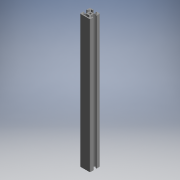
# Autodesk Inventor part: NFSF5-2020-263.5
Saved by Autodesk Inventor 2017.3 (Build 213256000, 256)
## iProperties
Part Number: NFSF5-2020-263.5
Material: Generic
Catalog Web Link: www.cadenas.de
Description: NFS5-2020, NFSB5-2020, HFS5-2020, HFSB5-2020, CAF5-2020, HFSY5-2020, NFSF5-2020, HFSF5-2020, HFSFB5-2020, NFST5-2020, HFST5-2020, HFSTB5-2020, HFSH5-2020, HFSC5-2020-HFS5 Series Aluminum Extrusions 20 Square -1 Slot-
Vendor: MISUMI
Document SubType Name: Modeling
Designer: partserver
Manufacturer: MISUMI
Mass: 51.0572 g
Surface Area: 481.65 cm^2
Volume: 51.0572 cm^3
Density: 1 g/cm^3
Appearance: PSOLRGB-175-175-175
Category: PARTsolutions
Company: MISUMI
Title: NFSF5-2020-263.5
Author: Cadenas PARTsolutions
Comments: HFS5 Series Aluminum Extrusions 20 Square -1 Slot-
PSOL_IDENT_0: {$CADENAS_DATA\23d-libs\misumi\metric\38_al_extrusions_blackets\5\hfs5_2020.prj},682 {VTYP=3D},{NB=N
PSOL_IDENT_1: FSF5-2020-263.5},{LINA=NFSF5-2020-263.5},{NN=NFS5-2020, NFSB5-2020, HFS5-2020, HFSB5-2020, CAF5-2020
PSOL_IDENT_2: , HFSY5-2020, NFSF5-2020, HFSF5-2020, HFSFB5-2020, NFST5-2020, HFST5-2020, HFSTB5-2020, HFSH5-2020,
PSOL_IDENT_3: HFSC5-2020},{DATE=09.09.2019 15:28:27},{GEOMDATE=18.06.2019 07:59:14},{VERSION=},{LINEID=40},{WBVAR=
PSOL_IDENT_4: L,ALT1,ALT2,ALT4,ALT5,CP5,DL5,DR5,ALT6,ALT9,ALT10,ALT11,HP6,NHL6,DL6,NHR6,DR6,ALT7,ALT8,NH9,AH,BH,CH
PSOL_IDENT_5: ,DH,EH,NH10,AV,BV,CV,DV,EV,NH11,AP,BP,CP,DP,EP,ALT12,ALT13,Z,NH12,XA,XB,XC,XD,XE,NH13,YA,YB,YC,YD,YE
PSOL_IDENT_6: ,ALT16,HP16,DL16,DR16,ALT17,HQ17,JLP,ALT20},{WBNUMERIC=L,NH9,AH,BH,CH,DH,EH,NH10,AV,BV,CV,DV,EV,NH11
PSOL_IDENT_7: ,AP,BP,CP,DP,EP,NH12,XA,XB,XC,XD,XE,NH13,YA,YB,YC,YD,YE,HQ17,JLP}  {NB=NFSF5-2020-263.5},{LINA=NFSF5
PSOL_IDENT_8: -2020-263.5},{KT=DUMMY},{PN=NFSF5-2020-263.5},{TPS=NFSF5-2020},{MAT=6063-T5 Aluminum Alloy},{ST=Clea
PSOL_IDENT_9: r Anodize},{FRMW=20},{FRMH=20},{FRD=4.2},{L=263.5},{MASS=0.53},{SA=195},{LX=0.834x10^4},{LY=0.746x10
PSOL_IDENT_10: ^4},{ALT1=},{M1=0},{DPL1=0},{DPR1=0},{ALT1PN=},{ALT2=},{ALT2ALG= '','w/o End Tapping (Heli-Coil Inse
PSOL_IDENT_11: rt)','LHP','with LHP (Tapping on the Left (Heli-Coil Insert))','RHP','with RHP (Tapping on the Right
PSOL_IDENT_12: (Heli-Coil Insert))','HPW','with HPW (Tapping on Both Ends (Heli-Coil Insert))' },{M2=0},{DP2=0},{A
PSOL_IDENT_13: LT2PN=},{ALT4=},{ALT4ALG= '', 'w/o SC (High Precision Cut)', 'SC', 'with SC (High Precision Cut)' },
PSOL_IDENT_14: {ALT4PN=},{ALT5=},{ALT5ALG= '','w/o 45 Degree Cut','1','with 45 Degree Cut' },{CP5=},{CP5ALG= '','N/
PSOL_IDENT_15: A' },{DL5=},{DL5ALG= '','N/A' },{DR5=},{DR5ALG= '','N/A' },{FRMLALT5=0},{FRMRALT5=0},{ALT5PN=},{ALT6=
PSOL_IDENT_16: },{ALT6ALG= '','w/o Fastening Location Wrench Access Hole Alterations','1','with Fastening Location
PSOL_IDENT_17: Wrench Access Hole Alterations' },{ALT9=},{ALT9ALG= '','w/o Location Specified Wrench Access Hole Al
PSOL_IDENT_18: teratons (Horizontal)','1','with Location Specified Wrench Access Hole Alteratons (Horizontal)' },{A
PSOL_IDENT_19: LT10=},{ALT10ALG= '','w/o Location Specified Wrench Access Hole Alteratons (Vertical)','1','with Loc
PSOL_IDENT_20: ation Specified Wrench Access Hole Alteratons (Vertical)' },{ALT11=},{ALT11ALG= '','w/o Location Spe
PSOL_IDENT_21: cified Wrench Access Hole Alteratons (Crisscross)','1','with Location Specified Wrench Access Hole A
PSOL_IDENT_22: lteratons (Crisscross)' },{HP6=},{HP6ALG= '','N/A' },{NHL6=},{NHL6ALG= '','N/A' },{DL6=},{DL6ALG= ''
PSOL_IDENT_23: ,'N/A' },{NHR6=},{NHR6ALG= '','N/A' },{DR6=},{DR6ALG= '','N/A' },{HL6=0.000},{HL6D=0},{HR6=0.000},{H
PSOL_IDENT_24: R6D=0},{J6=0},{J6D=0},{K6=0},{K6D=0},{DD6=0.00},{DD6ALG=0},{ALT7=},{ALT7ALG= '','N/A' },{ALT8=},{ALT
PSOL_IDENT_25: 8ALG= '','N/A' },{ALT678PN=},{NH9=0},{NH9MAX=5},{NH9ALG=[0]},{AH=0.0},{AHMIN=7},{AHMAX=258.5},{AHALG=
PSOL_IDENT_26: [0]},{BH=0.0},{BHMIN=2},{BHMAX=260.5},{BHALG=[0]},{CH=0.0},{CHMIN=2},{CHMAX=262.5},{CHALG=[0]},{DH=0
PSOL_IDENT_27: .0},{DHMIN=2},{DHMAX=264.5},{DHALG=[0]},{EH=0.0},{EHMIN=2},{EHMAX=256.5},{EHALG=[0]},{NH10=0},{NH10M
PSOL_IDENT_28: AX=5},{NH10ALG=[0]},{AV=0.0},{AVMIN=7},{AVMAX=258.5},{AVALG=[0]},{BV=0.0},{BVMIN=2},{BVMAX=260.5},{B
PSOL_IDENT_29: VALG=[0]},{CV=0.0},{CVMIN=2},{CVMAX=262.5},{CVALG=[0]},{DV=0.0},{DVMIN=2},{DVMAX=264.5},{DVALG=[0]},
PSOL_IDENT_30: {EV=0.0},{EVMIN=2},{EVMAX=256.5},{EVALG=[0]},{NH11=0},{NH11MAX=5},{NH11ALG=[0]},{AP=0.0},{APMIN=7},{
PSOL_IDENT_31: APMAX=258.5},{APALG=[0]},{BP=0.0},{BPMIN=2},{BPMAX=260.5},{BPALG=[0]},{CP=0.0},{CPMIN=2},{CPMAX=262.
PSOL_IDENT_32: 5},{CPALG=[0]},{DP=0.0},{DPMIN=2},{DPMAX=264.5},{DPALG=[0]},{EP=0.0},{EPMIN=2},{EPMAX=256.5},{EPALG=
PSOL_IDENT_33: [0]},{ALT9PN=},{ALT10PN=},{ALT11PN=},{ALT91011PN=},{ALT12=},{ALT12ALG= '','w/o Counterbore Hole in S
PSOL_IDENT_34: pecified Position (Vertical)','1','with Counterbore Hole in Specified Position (Vertical)' },{ALT13=
PSOL_IDENT_35: },{ALT13ALG= '','w/o Counterbore Hole in Specified Position (Horizontal)','1','with Counterbore Hole
PSOL_IDENT_36: in Specified Position (Horizontal)' },{Z=},{ZALG= '','N/A' },{DD12=0.0},{DD112=0.0},{NH12=0},{NH12M
PSOL_IDENT_37: AX=5},{NH12ALG=[0]},{XA=0.0},{XAMIN=7},{XAMAX=258.5},{XAALG=[0]},{XB=0.0},{XBMIN=2},{XBMAX=260.5},{X
PSOL_IDENT_38: BALG=[0]},{XC=0.0},{XCMIN=2},{XCMAX=262.5},{XCALG=[0]},{XD=0.0},{XDMIN=2},{XDMAX=264.5},{XDALG=[0]},
PSOL_IDENT_39: {XE=0.0},{XEMIN=2},{XEMAX=256.5},{XEALG=[0]},{NH13=0},{NH13MAX=5},{NH13ALG=[0]},{YA=0.0},{YAMIN=7},{
PSOL_IDENT_40: YAMAX=258.5},{YAALG=[0]},{YB=0.0},{YBMIN=2},{YBMAX=260.5},{YBALG=[0]},{YC=0.0},{YCMIN=2},{YCMAX=262.
PSOL_IDENT_41: 5},{YCALG=[0]},{YD=0.0},{YDMIN=2},{YDMAX=264.5},{YDALG=[0]},{YE=0.0},{YEMIN=2},{YEMAX=256.5},{YEALG=
PSOL_IDENT_42: [0]},{ALT12PN=},{ALT13PN=},{ALT1213PN=},{ALT16=},{ALT16ALG= '','w/o M Type Hole Alteration','1','wit
PSOL_IDENT_43: h M Type Hole Alteration' },{HP16=},{HP16ALG= '','N/A' },{DL16=},{DL16ALG= '','N/A' },{DR16=},{DR16A
PSOL_IDENT_44: LG= '','N/A' },{H116=0},{D16=0.0},{ALT16PN=},{ALT17=},{ALT17ALG= '','w/o L Type Hole Alteration (Top
PSOL_IDENT_45: )','1','with L Type Hole Alteration (Top)' },{HQ17=0},{HQ17ALG=0},{JLP=0},{JLPMIN=4.9},{JLPMAX=0},{J
PSOL_IDENT_46: LPALG=[0]},{L17=0},{D17=0.0},{ALT17PN=},{ALT20=},{ALT20PN=},{ERRORALT01=OK},{ERRORALT02=OK},{ERRORAL
PSOL_IDENT_47: T05=OK},{ERRORALT06091=OK},{ERRORALT06092=OK},{ERRORALT06093=OK},{ERRORALT06094=OK},{ERRORALT06101=O
PSOL_IDENT_48: K},{ERRORALT06102=OK},{ERRORALT06103=OK},{ERRORALT06104=OK},{ERRORALT06111=OK},{ERRORALT06112=OK},{E
PSOL_IDENT_49: RRORALT06113=OK},{ERRORALT06114=OK},{ERRORALT06121=OK},{ERRORALT06122=OK},{ERRORALT06123=OK},{ERRORA
PSOL_IDENT_50: LT06124=OK},{ERRORALT06131=OK},{ERRORALT06132=OK},{ERRORALT06133=OK},{ERRORALT06134=OK},{ERRORALT061
PSOL_IDENT_51: 6=OK},{ERRORALT06171=OK},{ERRORALT06172=OK},{ERRORALT06173=OK},{ERRORALT0911=OK},{ERRORALT0913=OK},{
PSOL_IDENT_52: ERRORALT0916=OK},{ERRORALT0917=OK},{ERRORALT1011=OK},{ERRORALT1012=OK},{ERRORALT1016=OK},{ERRORALT10
PSOL_IDENT_53: 17=OK},{ERRORALT1112=OK},{ERRORALT1113=OK},{ERRORALT1116=OK},{ERRORALT1117=OK},{ERRORALT1216=OK},{ER
PSOL_IDENT_54: RORALT1217=OK},{ERRORALT1316=OK},{ERRORALT1317=OK},{ERRORALT1617=OK},{ERRORPN=},{TFW=0}
NB: NFSF5-2020-263.5
NN: NFS5-2020, NFSB5-2020, HFS5-2020, HFSB5-2020, CAF5-2020, HFSY5-2020, NFSF5-2020, HFSF5-2020, HFSFB5-2020, NFST5-2020, HFST5-2020, HFSTB5-2020, HFSH5-2020, HFSC5-2020
NT: HFS5 Series Aluminum Extrusions 20 Square -1 Slot-
NBSYN: $PN.
LINA: NFSF5-2020-263.5
CATALOG: Misumi
PN: NFSF5-2020-263.5
TPS: NFSF5-2020
MAT: 6063-T5 Aluminum Alloy
ST: Clear Anodize
L: 263.5
MASS: 0.53
SA: 195
LX: 0.834x10^4
LY: 0.746x10^4
ALT1: w/o End Tapping
M1: 0
DPL1: 0
DPR1: 0
ALT2: w/o End Tapping (Heli-Coil Insert)
M2: 0
DP2: 0
ALT4: w/o SC (High Precision Cut)
ALT5: w/o 45 Degree Cut
CP5: N/A
DL5: N/A
DR5: N/A
ALT6: w/o Fastening Location Wrench Access Hole Alterations
ALT9: w/o Location Specified Wrench Access Hole Alteratons (Horizontal)
ALT10: w/o Location Specified Wrench Access Hole Alteratons (Vertical)
ALT11: w/o Location Specified Wrench Access Hole Alteratons (Crisscross)
HP6: N/A
NHL6: N/A
DL6: N/A
NHR6: N/A
DR6: N/A
HL6D: 0
HR6D: 0
J6D: 0
K6D: 0
DD6: 0
ALT7: N/A
ALT8: N/A
NH9: 0
AH: 0
BH: 0
CH: 0
DH: 0
EH: 0
NH10: 0
AV: 0
BV: 0
CV: 0
DV: 0
EV: 0
NH11: 0
AP: 0
BP: 0
CP: 0
DP: 0
EP: 0
ALT12: w/o Counterbore Hole in Specified Position (Vertical)
ALT13: w/o Counterbore Hole in Specified Position (Horizontal)
Z: N/A
DD12: 0
DD112: 0
NH12: 0
XA: 0
XB: 0
XC: 0
XD: 0
XE: 0
NH13: 0
YA: 0
YB: 0
YC: 0
YD: 0
YE: 0
ALT16: w/o M Type Hole Alteration
HP16: N/A
DL16: N/A
DR16: N/A
H116: 0
D16: 0
ALT17: w/o L Type Hole Alteration (Top)
HQ17: 0
JLP: 0
D17: 0
ALT20: w/o CW (End Face C Chamfering)
SUPPLIER: MISUMI
ARTICLENO: NFSF5-2020-263.5
BOMINFO: NFSF5-2020-263.5
CREATOR: CADENAS GmbH
Autodesk Inventor part; units mm, degrees
ref_plane "YZ Plane" through (0, 0, 0) normal (1, 0, 0) x (0, 1, 0)
ref_plane "XZ Plane" through (0, 0, 0) normal (0, 1, 0) x (-1, 0, 0)
ref_plane "XY Plane" through (0, 0, 0) normal (0, 0, 1) x (1, 0, 0)
sketch "Sketch_76" plane through (0, 0, 0) normal (0, 0, 1) x (1, 0, 0)
  line L0 (-10, -3) -> (-10, -9)
  arc A0 (-10, -9) -> (-9, -10) centre (-9, -9) ccw
  line L1 (-9, -10) -> (9, -10)
  arc A1 (9, -10) -> (10, -9) centre (9, -9) ccw
  line L2 (10, -9) -> (10, -3)
  line L3 (10, -3) -> (8, -3)
  line L4 (8, -3) -> (8, -6)
  line L5 (8, -6) -> (7.0607, -6)
  line L6 (7.0607, -6) -> (4, -2.9393)
  line L7 (4, -2.9393) -> (4, -0.6536)
  arc A2 (4, -0.6536) -> (3.933, -0.4036) centre (3.5, -0.6536) ccw
  line L8 (3.933, -0.4036) -> (3.7, 0)
  line L9 (3.7, 0) -> (3.933, 0.4036)
  arc A3 (3.933, 0.4036) -> (3.933, 0.9036) centre (3.5, 0.6536) ccw
  line L10 (3.933, 0.9036) -> (3.751, 1.2189)
  line L11 (3.751, 1.2189) -> (4, 2.5)
  line L12 (4, 2.5) -> (4, 2.9393)
  line L13 (4, 2.9393) -> (7.0607, 6)
  line L14 (7.0607, 6) -> (8, 6)
  line L15 (8, 6) -> (8, 3)
  line L16 (8, 3) -> (10, 3)
  line L17 (10, 3) -> (10, 9)
  arc A4 (10, 9) -> (9, 10) centre (9, 9) ccw
  line L18 (9, 10) -> (3, 10)
  line L19 (3, 10) -> (3, 8)
  line L20 (3, 8) -> (6, 8)
  line L21 (6, 8) -> (6, 7.0607)
  line L22 (6, 7.0607) -> (2.9393, 4)
  line L23 (2.9393, 4) -> (0.6536, 4)
  arc A5 (0.6536, 4) -> (0.4036, 3.933) centre (0.6536, 3.5) ccw
  line L24 (0.4036, 3.933) -> (0, 3.7)
  line L25 (0, 3.7) -> (-0.4036, 3.933)
  arc A6 (-0.4036, 3.933) -> (-0.9036, 3.933) centre (-0.6536, 3.5) ccw
  line L26 (-0.9036, 3.933) -> (-1.2189, 3.751)
  line L27 (-1.2189, 3.751) -> (-2.5, 4)
  line L28 (-2.5, 4) -> (-2.9393, 4)
  line L29 (-2.9393, 4) -> (-6, 7.0607)
  line L30 (-6, 7.0607) -> (-6, 8)
  line L31 (-6, 8) -> (-3, 8)
  line L32 (-3, 8) -> (-3, 10)
  line L33 (-3, 10) -> (-9, 10)
  arc A7 (-9, 10) -> (-10, 9) centre (-9, 9) ccw
  line L34 (-10, 9) -> (-10, 3)
  line L35 (-10, 3) -> (-8, 3)
  line L36 (-8, 3) -> (-8, 6)
  line L37 (-8, 6) -> (-7.0607, 6)
  line L38 (-7.0607, 6) -> (-4, 2.9393)
  line L39 (-4, 2.9393) -> (-4, 0.6536)
  arc A8 (-4, 0.6536) -> (-3.933, 0.4036) centre (-3.5, 0.6536) ccw
  line L40 (-3.933, 0.4036) -> (-3.7, 0)
  line L41 (-3.7, 0) -> (-3.933, -0.4036)
  arc A9 (-3.933, -0.4036) -> (-3.933, -0.9036) centre (-3.5, -0.6536) ccw
  line L42 (-3.933, -0.9036) -> (-3.751, -1.2189)
  line L43 (-3.751, -1.2189) -> (-4, -2.5)
  line L44 (-4, -2.5) -> (-4, -2.9393)
  line L45 (-4, -2.9393) -> (-7.0607, -6)
  line L46 (-7.0607, -6) -> (-8, -6)
  line L47 (-8, -6) -> (-8, -3)
  line L48 (-8, -3) -> (-10, -3)
  line L49 (-6, -7.2678) -> (-6, -7.5)
  arc A10 (-6, -7.5) -> (-5.5, -8) centre (-5.5, -7.5) ccw
  line L50 (-5.5, -8) -> (5.5, -8)
  arc A11 (5.5, -8) -> (6, -7.5) centre (5.5, -7.5) ccw
  line L51 (6, -7.5) -> (6, -7.2678)
  arc A12 (6, -7.2678) -> (5.8536, -6.9142) centre (5.5, -7.2678) ccw
  line L52 (5.8536, -6.9142) -> (3.0858, -4.1464)
  arc A13 (3.0858, -4.1464) -> (2.7322, -4) centre (2.7322, -4.5) ccw
  line L53 (2.7322, -4) -> (-2.7322, -4)
  arc A14 (-2.7322, -4) -> (-3.0858, -4.1464) centre (-2.7322, -4.5) ccw
  line L54 (-3.0858, -4.1464) -> (-5.8536, -6.9142)
  arc A15 (-5.8536, -6.9142) -> (-6, -7.2678) centre (-5.5, -7.2678) ccw
  constraints: 110 end point, 32 point on circle, 16 centre point
extrude "Extrusion1" add sketch "Sketch_76" against normal blind 263.5
sketch "Sketch2" plane through (0, 0, -263.5) normal (0, 0, -1) x (-1, 0, 0)
  point P0 (0, 0)
hole "Hole1" at (0, 0, -263.5) direction (0, 0, 1) diameter 4.2 depth 263.5
ref_plane "C1_XY" through (0, 0, 0) normal (0, 0, 1) x (1, 0, 0)
ref_plane "C1_YZ" through (0, 0, 0) normal (1, 0, 0) x (0, 1, 0)
ref_plane "C1_ZX" through (0, 0, 0) normal (0, 1, 0) x (0, 0, 1)
body "Solid1"
